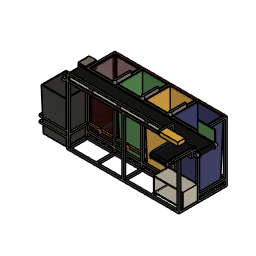
e-waste v4 ATOM (Autodesk Fusion 360 design; units mm, degrees)
Autodesk Fusion 360 part; units mm, degrees
(part 1 of 3)
sketch "Sketch1" plane through (0, 0, 0) normal (0, 0, 1) x (1, 0, 0)
sketch "Sketch1 (2)" plane through (0, 0, 0) normal (0, 0, 1) x (1, 0, 0) in component "belt sensor"
  line L0 (1400, -450) -> (1200, -450)
  line L1 (1200, -450) -> (1200, -800)
  line L2 (1200, -800) -> (1400, -800)
  line L3 (1400, -800) -> (1400, -450)
  constraint horizontal L0
  constraint perpendicular L0 L1
  constraint perpendicular L1 L2
  constraint perpendicular L0 L3
extrude "Extrude1" add sketch "Sketch1 (2)" along normal blind 70 makes body 1 in component "belt sensor"
sketch "Sketch2" plane through (1400, 0, 0) normal (1, 0, 0) x (0, 1, 0) in component "belt sensor"
sketch "Sketch3" plane through (1400, 0, 0) normal (1, 0, 0) x (0, 1, 0) in component "belt sensor"
sketch "Sketch4" plane through (1400, 0, 0) normal (1, 0, 0) x (0, 1, 0) in component "belt sensor"
  circle A0 centre (-800, 35) radius 35
  circle A1 centre (-800, 35) radius 30
  constraint concentric A0 A1
extrude "Extrude2" add sketch "Sketch4" against normal blind 200 bodies 1 in component "belt sensor"
sketch "Sketch5" plane through (1400, 0, 0) normal (1, 0, 0) x (0, 1, 0) in component "belt sensor"
  circle A0 centre (-450, 35) radius 35
  circle A1 centre (-450, 35) radius 30
  constraint concentric A0 A1
extrude "Extrude3" add sketch "Sketch5" against normal blind 200 bodies 1 in component "belt sensor"
sketch "Sketch6" plane through (1400, 0, 0) normal (1, 0, 0) x (0, 1, 0) in component "belt sensor"
  line L0 (-800, 65) -> (-450, 65)
  line L1 (-450, 65) -> (-450, 5)
  line L2 (-450, 5) -> (-800, 5)
  line L3 (-800, 5) -> (-800, 65)
  constraint horizontal L0
  constraint vertical L1
  constraint horizontal L2
  constraint vertical L3
extrude "Extrude4" cut sketch "Sketch6" against normal blind 300 bodies 1 in component "belt sensor"
sketch "Sketch7" plane through (1400, 0, 0) normal (1, 0, 0) x (0, 1, 0) in component "belt sensor"
  line L0 (-450, 5) -> (-800, 5)
  arc A0 (-800, 65) -> (-800, 5) centre (-800, 35) ccw
  line L1 (-800, 65) -> (-450, 65)
  arc A1 (-450, 5) -> (-450, 65) centre (-450, 35) ccw
  arc A2 (-450, 0) -> (-450, 70) centre (-450, 35) ccw
  line L2 (-450, 70) -> (-800, 70)
  arc A3 (-800, 70) -> (-800, 0) centre (-800, 35) ccw
  line L3 (-800, 0) -> (-450, 0)
  circle A4 centre (-800, 35) radius 27.5
  dimension "d42" = 55
  constraint concentric A0 A4
  measures "d42" diameter of A4
extrude "Extrude5" add sketch "Sketch7" against normal blind 200 separate body contours A4 makes body 2 in component "belt sensor"
sketch "Sketch8" plane through (1400, 0, 0) normal (1, 0, 0) x (0, 1, 0) in component "belt sensor"
  circle A0 centre (-800, 35) radius 27.5
  circle A1 centre (-450, 35) radius 27.5
  dimension "d45" = 55
  measures "d45" diameter of A1
extrude "Extrude6" add sketch "Sketch8" against normal blind 200 separate body contours A1 makes body 3 in component "belt sensor"
move_body "Move1" bodies 2 3 1 to x (1, 0, 0) y (0, 1, 0) z (0, 0, 1) at (0, 180, 750) in component "belt sensor"
move_body "Move2" bodies 2 3 1 to x (1, 0, 0) y (0, 1, 0) z (0, 0, 1) at (200, 0, 0) in component "belt sensor"
sketch "Sketch1 (3)" plane through (0, 0, 0) normal (0, 1, 0) x (1, 0, 0) in component "belt"
  line L0 (0, 500) -> (1800, 500)
  line L1 (1800, 500) -> (1800, 430)
  line L2 (1800, 430) -> (0, 430)
  line L3 (0, 430) -> (0, 500)
  dimension "d68" = 1800
  dimension "d69" = 70
  constraint horizontal L0
  constraint perpendicular L0 L1
  constraint perpendicular L1 L2
  constraint perpendicular L0 L3
  measures "d68" distance of L0.start L0.end
  measures "d69" distance of L0.end L1.end
extrude "Extrude1'" add sketch "Sketch1 (3)" along normal blind 200 separate body makes body 4 in component "belt"
sketch "Sketch2 (2)" plane through (0, 0, 0) normal (0, -1, 0) x (1, 0, 0) in component "belt"
  line L0 (1800, -430) -> (0, -430)
  line L1 (0, -430) -> (0, -500)
  line L2 (0, -500) -> (1800, -500)
  line L3 (1800, -500) -> (1800, -430)
  circle A0 centre (0, -465) radius 35
  circle A1 centre (0, -465) radius 30
  dimension "d72" = 60
  constraint midpoint L1 A0.centre
  constraint coincident L0.end A0
  constraint concentric A0 A1
  measures "d72" diameter of A1
extrude "Extrude2'" add sketch "Sketch2 (2)" against normal blind 200 contours L1 A0 A1 picked at (-12.8396, -434.3307) bodies 4 in component "belt"
sketch "Sketch3 (2)" plane through (0, 0, 0) normal (0, -1, 0) x (1, 0, 0) in component "belt"
  line L0 (0, -500) -> (1800, -500)
  line L1 (1800, -500) -> (1800, -430)
  line L2 (1800, -430) -> (0, -430)
  arc A0 (0, -430) -> (0, -500) centre (0, -465) ccw
  arc A1 (0, -435) -> (0, -495) centre (0, -465) ccw
  line L3 (0, -435) -> (0, -495)
  circle A2 centre (1800, -465) radius 35
  circle A3 centre (1800, -465) radius 30
  dimension "d75" = 60
  constraint midpoint L1 A2.centre
  constraint coincident L1.end A2
  constraint concentric A2 A3
  measures "d75" diameter of A3
extrude "Extrude3'" add sketch "Sketch3 (2)" against normal blind 200 contours L1 A2 A3 picked at (1831.4014, -454.0493) bodies 4 in component "belt"
sketch "Sketch4 (2)" plane through (0, 0, 0) normal (0, -1, 0) x (1, 0, 0) in component "belt"
  line L0 (1800, -430) -> (0, -430)
  arc A0 (0, -430) -> (0, -500) centre (0, -465) ccw
  line L1 (0, -500) -> (1800, -500)
  arc A1 (1800, -500) -> (1800, -430) centre (1800, -465) ccw
  arc A2 (1800, -495) -> (1800, -435) centre (1800, -465) ccw
  line L2 (1800, -495) -> (1800, -435)
  arc A3 (0, -435) -> (0, -495) centre (0, -465) ccw
  line L3 (0, -435) -> (0, -495)
  line L4 (0, -435) -> (1800, -435)
  line L5 (1800, -435) -> (1800, -495)
  line L6 (1800, -495) -> (0, -495)
  line L7 (0, -495) -> (0, -435)
  constraint horizontal L4
  constraint vertical L5
  constraint horizontal L6
  constraint vertical L7
  constraint coincident A2.start L2.start
  constraint coincident A3.start L3.start
extrude "Extrude4'" cut sketch "Sketch4 (2)" against normal blind 300 contours L2 L3 L4 L5 L6 L7 bodies 4 in component "belt"
sketch "Sketch5 (2)" plane through (0, 0, 0) normal (0, -1, 0) x (1, 0, 0) in component "belt"
  line L0 (0, -435) -> (1800, -435)
  arc A0 (1800, -495) -> (1800, -435) centre (1800, -465) ccw
  line L1 (1800, -495) -> (0, -495)
  arc A1 (0, -435) -> (0, -495) centre (0, -465) ccw
  line L2 (1800, -430) -> (0, -430)
  arc A2 (0, -430) -> (0, -500) centre (0, -465) ccw
  line L3 (0, -500) -> (1800, -500)
  arc A3 (1800, -500) -> (1800, -430) centre (1800, -465) ccw
  circle A4 centre (0, -465) radius 27.5
  circle A5 centre (1800, -465) radius 27.5
  dimension "d80" = 55
  dimension "d81" = 55
  constraint concentric A1 A4
  constraint concentric A0 A5
  measures "d80" diameter of A4
  measures "d81" diameter of A5
extrude "Extrude5'" add sketch "Sketch5 (2)" against normal blind 200 separate body contours A4 | A5 makes body 5 at (27.3633, 66.6667, -467.7381) makes body 6 at (1816.053, 133.3333, -442.6717) in component "belt"
move_body "Move1'" bodies 5 4 6 to x (1, 0, 0) y (0, 1, 0) z (0, 0, 1) at (0, -225, 1250) in component "belt"
move_body "Move2'" bodies 5 4 6 to x (1, 0, 0) y (0, 1, 0) z (0, 0, 1) at (-160, 0, 0) in component "belt"
sketch "Sketch1 (4)" plane through (0, 0, 0) normal (0, 1, 0) x (1, 0, 0) in component "power"
  line L0 (1500, 0) -> (1100, 0)
  line L1 (1100, 0) -> (1100, -200)
  line L2 (1100, -200) -> (1500, -200)
  line L3 (1500, -200) -> (1500, 0)
  dimension "d313" = 400
  constraint horizontal L0
  constraint perpendicular L0 L1
  constraint perpendicular L1 L2
  constraint perpendicular L0 L3
  measures "d313" distance of L1 L3
extrude "Extrude1''" add sketch "Sketch1 (4)" against normal blind 200 separate body makes body 7 in component "power"
sketch "Sketch2 (3)" plane through (0, -200, 0) normal (0, -1, 0) x (1, 0, 0) in component "power"
  line L0 (1500, 0) -> (1500, 200)
  line L1 (1500, 200) -> (1100, 200)
  line L2 (1100, 200) -> (1100, 0)
  line L3 (1100, 0) -> (1500, 0)
  line L4 (1110, 190) -> (1490, 190)
  line L5 (1490, 190) -> (1490, 10)
  line L6 (1490, 10) -> (1110, 10)
  line L7 (1110, 10) -> (1110, 190)
  dimension "d314" = 10
  dimension "d315" = 10
  dimension "d316" = 10
  dimension "d317" = 10
  constraint perpendicular L0 L4
  constraint perpendicular L4 L5
  constraint perpendicular L5 L6
  constraint perpendicular L4 L7
  measures "d314" distance of L0 L5
  measures "d315" distance of L2 L7
  measures "d316" distance of L1 L4
  measures "d317" distance of L3 L6
extrude "Extrude2''" cut sketch "Sketch2 (3)" against normal blind 190 contours L4 L5 L6 L7 bodies 7 in component "power"
sketch "Sketch2 (4)" plane through (0, 0, 0) normal (0, 0, 1) x (1, 0, 0)
sketch "Sketch1 (5)" plane through (0, 0, 0) normal (0, 0, 1) x (1, 0, 0) in component "vibrator"
  line L0 (0, 850) -> (200, 850)
  line L1 (200, 850) -> (200, 1050)
  line L2 (200, 1050) -> (0, 1050)
  line L3 (0, 1050) -> (0, 850)
  dimension "d89" = 200
  dimension "d90" = 200
  constraint horizontal L0
  constraint perpendicular L0 L1
  constraint perpendicular L1 L2
  constraint perpendicular L0 L3
  measures "d89" distance of L0.start L0.end
  measures "d90" distance of L0.end L1.end
sketch "Sketch1 (6)" plane through (0, 0, 0) normal (0, 0, 1) x (1, 0, 0) in component "bin case"
  line L0 (-109.9325, 100) -> (-459.9325, 100)
  line L1 (-459.9325, 100) -> (-459.9325, 450)
  line L2 (-459.9325, 450) -> (-109.9325, 450)
  line L3 (-109.9325, 450) -> (-109.9325, 100)
  line L4 (-84.9325, 450) -> (265.0675, 450)
  line L5 (265.0675, 450) -> (265.0675, 100)
  line L6 (265.0675, 100) -> (-84.9325, 100)
  line L7 (-84.9325, 100) -> (-84.9325, 450)
  line L8 (-84.9325, 100) -> (-84.9325, 450)
  line L9 (290.0675, 450) -> (640.0675, 450)
  line L10 (640.0675, 450) -> (640.0675, 100)
  line L11 (640.0675, 100) -> (290.0675, 100)
  line L12 (290.0675, 100) -> (290.0675, 450)
  line L13 (665.0675, 450) -> (1015.0675, 450)
  line L14 (1015.0675, 450) -> (1015.0675, 100)
  line L15 (1015.0675, 100) -> (665.0675, 100)
  line L16 (665.0675, 100) -> (665.0675, 450)
  line L17 (-484.9325, 475) -> (1040.0675, 475)
  line L18 (1040.0675, 475) -> (1040.0675, 75)
  line L19 (1040.0675, 75) -> (-484.9325, 75)
  line L20 (-484.9325, 75) -> (-484.9325, 475)
  dimension "d101" = 350
  dimension "d102" = 350
  dimension "d103" = 350
  dimension "d104" = 25
  dimension "d105" = 25
  dimension "d106" = 25
  dimension "d107" = 350
  dimension "d108" = 350
  dimension "d109" = 25
  dimension "d110" = 25
  dimension "d111" = 25
  dimension "d112" = 25
  constraint horizontal L0
  constraint vertical L1
  constraint horizontal L2
  constraint vertical L3
  constraint horizontal L4
  constraint vertical L5
  constraint horizontal L6
  constraint vertical L7
  constraint vertical L8
  constraint horizontal L9
  constraint vertical L10
  constraint horizontal L11
  constraint vertical L12
  constraint horizontal L13
  constraint vertical L14
  constraint horizontal L15
  constraint vertical L16
  constraint horizontal L17
  constraint vertical L18
  constraint horizontal L19
  constraint vertical L20
  measures "d101" distance of L0.start L0.end
  measures "d102" distance of L5.end L6.end
  measures "d103" distance of L10.end L11.end
  measures "d104" distance of L5 L12
  measures "d105" distance of L3 L7
  measures "d106" distance of L10 L16
  measures "d107" distance of L14.end L15.end
  measures "d108" distance of L0.end L1.end
  measures "d109" distance of L1 L20
  measures "d110" distance of L14 L18
  measures "d111" distance of L13 L17
  measures "d112" distance of L15 L19
extrude "Extrude1'''" add sketch "Sketch1 (6)" along normal blind 25 separate body makes body 8 in component "bin case"
sketch "Sketch1 (7)" plane through (0, 0, 0) normal (0, 0, 1) x (1, 0, 0) in component "bin case (1)"
  line L0 (-109.9325, 100) -> (-459.9325, 100)
  line L1 (-459.9325, 100) -> (-459.9325, 450)
  line L2 (-459.9325, 450) -> (-109.9325, 450)
  line L3 (-109.9325, 450) -> (-109.9325, 100)
  line L4 (-84.9325, 450) -> (265.0675, 450)
  line L5 (265.0675, 450) -> (265.0675, 100)
  line L6 (265.0675, 100) -> (-84.9325, 100)
  line L7 (-84.9325, 100) -> (-84.9325, 450)
  line L8 (-84.9325, 100) -> (-84.9325, 450)
  line L9 (290.0675, 450) -> (640.0675, 450)
  line L10 (640.0675, 450) -> (640.0675, 100)
  line L11 (640.0675, 100) -> (290.0675, 100)
  line L12 (290.0675, 100) -> (290.0675, 450)
  line L13 (665.0675, 450) -> (1015.0675, 450)
  line L14 (1015.0675, 450) -> (1015.0675, 100)
  line L15 (1015.0675, 100) -> (665.0675, 100)
  line L16 (665.0675, 100) -> (665.0675, 450)
  line L17 (-484.9325, 475) -> (1040.0675, 475)
  line L18 (1040.0675, 475) -> (1040.0675, 75)
  line L19 (1040.0675, 75) -> (-484.9325, 75)
  line L20 (-484.9325, 75) -> (-484.9325, 475)
  dimension "d101_1" = 350
  dimension "d102_1" = 350
  dimension "d103_1" = 350
  dimension "d104_1" = 25
  dimension "d105_1" = 25
  dimension "d106_1" = 25
  dimension "d107_1" = 350
  dimension "d108_1" = 350
  dimension "d109_1" = 25
  dimension "d110_1" = 25
  dimension "d111_1" = 25
  dimension "d112_1" = 25
  constraint horizontal L0
  constraint vertical L1
  constraint horizontal L2
  constraint vertical L3
  constraint horizontal L4
  constraint vertical L5
  constraint horizontal L6
  constraint vertical L7
  constraint vertical L8
  constraint horizontal L9
  constraint vertical L10
  constraint horizontal L11
  constraint vertical L12
  constraint horizontal L13
  constraint vertical L14
  constraint horizontal L15
  constraint vertical L16
  constraint horizontal L17
  constraint vertical L18
  constraint horizontal L19
  constraint vertical L20
  measures "d101_1" distance of L0.start L0.end
  measures "d102_1" distance of L5.end L6.end
  measures "d103_1" distance of L10.end L11.end
  measures "d104_1" distance of L5 L12
  measures "d105_1" distance of L3 L7
  measures "d106_1" distance of L10 L16
  measures "d107_1" distance of L14.end L15.end
  measures "d108_1" distance of L0.end L1.end
  measures "d109_1" distance of L1 L20
  measures "d110_1" distance of L14 L18
  measures "d111_1" distance of L13 L17
  measures "d112_1" distance of L15 L19
extrude "Extrude1''''" add sketch "Sketch1 (7)" along normal blind 25 separate body makes body 9 in component "bin case (1)"
sketch "Sketch3 (3)" plane through (0, 0, 25) normal (0, 0, 1) x (-1, 0, 0)
  line L0 (-265.0675, -100) -> (84.9325, -100)
  line L1 (84.9325, -100) -> (84.9325, -450)
  line L2 (84.9325, -450) -> (-265.0675, -450)
  line L3 (-265.0675, -450) -> (-265.0675, -100)
  line L4 (459.9325, -450) -> (109.9325, -450)
  line L5 (109.9325, -450) -> (109.9325, -100)
  line L6 (109.9325, -100) -> (459.9325, -100)
  line L7 (459.9325, -100) -> (459.9325, -450)
  line L8 (-640.0675, -100) -> (-290.0675, -100)
  line L9 (-290.0675, -100) -> (-290.0675, -450)
  line L10 (-290.0675, -450) -> (-640.0675, -450)
  line L11 (-640.0675, -450) -> (-640.0675, -100)
  line L12 (-1015.0675, -100) -> (-665.0675, -100)
  line L13 (-665.0675, -100) -> (-665.0675, -450)
  line L14 (-665.0675, -450) -> (-1015.0675, -450)
  line L15 (-1015.0675, -450) -> (-1015.0675, -100)
  line L16 (484.9325, -75) -> (-1040.0675, -75)
  line L17 (-1040.0675, -75) -> (-1040.0675, -475)
  line L18 (-1040.0675, -475) -> (484.9325, -475)
  line L19 (484.9325, -475) -> (484.9325, -75)
  line L20 (459.9325, -450) -> (484.9325, -450)
  line L21 (484.9325, -450) -> (484.9325, -475)
  line L22 (484.9325, -475) -> (459.9325, -475)
  line L23 (459.9325, -475) -> (459.9325, -450)
  line L24 (84.9325, -450) -> (109.9325, -450)
  line L25 (109.9325, -450) -> (109.9325, -475)
  line L26 (84.9325, -475) -> (84.9325, -450)
  line L27 (109.9325, -475) -> (84.9325, -475)
  line L28 (-290.0675, -450) -> (-265.0675, -450)
  line L29 (-265.0675, -450) -> (-265.0675, -475)
  line L30 (-290.0675, -475) -> (-290.0675, -450)
  line L31 (-265.0675, -475) -> (-290.0675, -475)
  line L32 (-665.0675, -450) -> (-640.0675, -450)
  line L33 (-640.0675, -450) -> (-640.0675, -475)
  line L34 (-665.0675, -475) -> (-665.0675, -450)
  line L35 (-640.0675, -475) -> (-665.0675, -475)
  line L36 (-1040.0675, -450) -> (-1015.0675, -450)
  line L37 (-1015.0675, -450) -> (-1015.0675, -475)
  line L38 (-1040.0675, -475) -> (-1040.0675, -450)
  line L39 (-1015.0675, -475) -> (-1040.0675, -475)
  line L40 (459.9325, -75) -> (484.9325, -75)
  line L41 (484.9325, -75) -> (484.9325, -100)
  line L42 (459.9325, -100) -> (459.9325, -75)
  line L43 (484.9325, -100) -> (459.9325, -100)
  line L44 (84.9325, -75) -> (109.9325, -75)
  line L45 (109.9325, -75) -> (109.9325, -100)
  line L46 (84.9325, -100) -> (84.9325, -75)
  line L47 (109.9325, -100) -> (84.9325, -100)
  line L48 (-290.0675, -75) -> (-265.0675, -75)
  line L49 (-265.0675, -75) -> (-265.0675, -100)
  line L50 (-290.0675, -100) -> (-290.0675, -75)
  line L51 (-265.0675, -100) -> (-290.0675, -100)
  line L52 (-665.0675, -75) -> (-640.0675, -75)
  line L53 (-640.0675, -75) -> (-640.0675, -100)
  line L54 (-665.0675, -100) -> (-665.0675, -75)
  line L55 (-640.0675, -100) -> (-665.0675, -100)
  line L56 (-1040.0675, -75) -> (-1015.0675, -75)
  line L57 (-1015.0675, -75) -> (-1015.0675, -100)
  line L58 (-1040.0675, -100) -> (-1040.0675, -75)
  line L59 (-1015.0675, -100) -> (-1040.0675, -100)
  dimension "d117" = -1500
  dimension "d118" = 375
  constraint horizontal L20
  constraint vertical L21
  constraint horizontal L22
  constraint vertical L23
  constraint coincident L18.end L19.start
  constraint coincident L4.start L7.end
move_body "Move1''" bodies 8 to x (1, 0, 0) y (0, 1, 0) z (0, 0, 1) at (0, 0, 800) in component "bin case"
extrude "Extrude2'''" add sketch "Sketch3 (3)" along normal blind 775 contours L16 L48 L49 L50 L51 | L16 L44 L45 L46 L47 | L18 L28 L29 L30 L31 | L18 L24 L25 L26 L27 | L16 L52 L53 L54 L55 | L16 L19 L40 L41 L42 L43 | L18 L32 L33 L34 L35 | L18 L19 L20 L21 L22 L23 | L16 L17 L56 L57 L58 L59 | L17 L18 L36 L37 L38 L39 bodies 8 in component "bin case"
combine "Combine1" operation add target body 9 tool bodies 8 in component "bin case (1)"
sketch "Sketch4 (3)" plane through (-459.9325, 0, 0) normal (1, 0, 0) x (0, 1, 0)
  line L0 (100, 0) -> (450, 0)
  line L1 (450, 0) -> (450, 25)
  line L2 (450, 25) -> (100, 25)
  line L3 (100, 25) -> (100, 0)
sketch "Sketch5 (3)" plane through (-459.9325, 275, 12.5) normal (1, 0, 0) x (0, 1, 0)
sketch "Sketch6 (2)" plane through (1040.0675, 0, 0) normal (1, 0, 0) x (0, 1, 0)
  line L0 (75, 825) -> (75, 0)
  line L1 (75, 0) -> (475, 0)
  line L2 (475, 0) -> (475, 825)
  line L3 (475, 825) -> (75, 825)
  line L4 (100, 25) -> (100, 800)
  line L5 (100, 800) -> (450, 800)
  line L6 (450, 800) -> (450, 25)
  line L7 (450, 25) -> (100, 25)
  line L8 (200, 25) -> (225, 25)
  line L9 (225, 25) -> (225, 0)
  line L10 (225, 0) -> (200, 0)
  line L11 (200, 0) -> (200, 25)
  line L12 (325, 25) -> (350, 25)
  line L13 (350, 25) -> (350, 0)
  line L14 (350, 0) -> (325, 0)
  line L15 (325, 0) -> (325, 25)
  dimension "d121" = 25
  dimension "d122" = 25
  dimension "d123" = 100
  dimension "d124" = 100
  constraint horizontal L8
  constraint vertical L9
  constraint horizontal L10
  constraint vertical L11
  constraint coincident L7 L8.start
  constraint horizontal L12
  constraint vertical L13
  constraint horizontal L14
  constraint vertical L15
  constraint coincident L7 L12.start
  measures "d121" distance of L8.start L8.end
  measures "d122" distance of L12.start L12.end
  measures "d123" distance of L4 L11
  measures "d124" distance of L6 L13
extrude "Extrude2''''" add sketch "Sketch6 (2)" against normal blind 1525 contours L1 L7 L8 L9 L10 L11 | L1 L7 L12 L13 L14 L15 bodies 9 in component "bin case (1)"
sketch "Sketch7 (2)" plane through (0, 75, 0) normal (0, -1, 0) x (1, 0, 0)
  line L0 (1015.0675, 25) -> (665.0675, 25)
  line L1 (665.0675, 25) -> (665.0675, 800)
  line L2 (665.0675, 800) -> (1015.0675, 800)
  line L3 (1015.0675, 800) -> (1015.0675, 25)
  line L4 (265.0675, 25) -> (-84.9325, 25)
  line L5 (-84.9325, 25) -> (-84.9325, 800)
  line L6 (-84.9325, 800) -> (265.0675, 800)
  line L7 (265.0675, 800) -> (265.0675, 25)
  line L8 (1040.0675, 0) -> (1040.0675, 825)
  line L9 (1040.0675, 825) -> (-484.9325, 825)
  line L10 (-484.9325, 825) -> (-484.9325, 0)
  line L11 (-484.9325, 0) -> (1040.0675, 0)
  line L12 (-459.9325, 25) -> (-459.9325, 800)
  line L13 (-459.9325, 800) -> (-109.9325, 800)
  line L14 (-109.9325, 800) -> (-109.9325, 25)
  line L15 (-109.9325, 25) -> (-459.9325, 25)
  line L16 (290.0675, 25) -> (290.0675, 800)
  line L17 (290.0675, 800) -> (640.0675, 800)
  line L18 (640.0675, 800) -> (640.0675, 25)
  line L19 (640.0675, 25) -> (290.0675, 25)
sketch "Sketch8 (2)" plane through (0, 75, 0) normal (0, -1, 0) x (1, 0, 0)
  line L0 (-485, 875) -> (-585, 875)
  line L1 (-585, 875) -> (-585, 775)
  line L2 (-585, 775) -> (-485, 775)
  line L3 (-485, 775) -> (-485, 875)
  line L4 (1040.0675, 825) -> (-484.9325, 825)
  line L5 (-575, 865) -> (-495, 865)
  line L6 (-495, 865) -> (-495, 785)
  line L7 (-495, 785) -> (-575, 785)
  line L8 (-575, 785) -> (-575, 865)
  dimension "d133" = 100
  dimension "d134" = 100
  dimension "d135" = 50
  dimension "d136" = 10
  dimension "d137" = 10
  dimension "d138" = 10
  dimension "d139" = 10
  constraint horizontal L0
  constraint vertical L1
  constraint horizontal L2
  constraint vertical L3
  constraint horizontal L5
  constraint vertical L6
  constraint horizontal L7
  constraint vertical L8
  measures "d133" distance of L0.start L0.end
  measures "d134" distance of L0.end L1.end
  measures "d135" distance of L0 L4
  measures "d136" distance of L1 L8
  measures "d137" distance of L3 L6
  measures "d138" distance of L2 L7
  measures "d139" distance of L0 L5
extrude "Extrude1'''''" add sketch "Sketch8 (2)" against normal blind 150 separate body makes body 10
copy_body "CutPasteBodies1" bodies 10 removing the originals makes body 11 in component "motor belt"
sketch "Sketch1 (8)" plane through (0, 75, 0) normal (0, -1, 0) x (1, 0, 0) in component "motor belt"
  line L0 (-495, 785) -> (-575, 785)
  line L1 (-575, 785) -> (-575, 865)
  line L2 (-575, 865) -> (-495, 865)
  line L3 (-495, 865) -> (-495, 785)
  line L4 (-485, 775) -> (-485, 875)
  line L5 (-485, 875) -> (-585, 875)
  line L6 (-585, 875) -> (-585, 775)
  line L7 (-585, 775) -> (-485, 775)
  circle A0 centre (-535, 825) radius 40
  constraint tangent L0 A0
extrude "Extrude1''''''" add sketch "Sketch1 (8)" against normal blind 100 separate body contours A0 makes body 12 in component "motor belt"
sketch "Sketch2 (5)" plane through (0, 75, 0) normal (0, -1, 0) x (1, 0, 0) in component "motor belt"
  circle A0 centre (-535, 825) radius 40
  circle A1 centre (-535, 825) radius 20
  dimension "d144" = 40
  constraint concentric A0 A1
  measures "d144" diameter of A1
extrude "Extrude2'''''" add sketch "Sketch2 (5)" along normal blind 20 contours A1 bodies 12 in component "motor belt"
move_body "Move1'''" bodies 12 11 to x (1, 0, 0) y (0, 1, 0) z (0, 0, 1) at (0, 0, -30) in component "motor belt"
sketch "Sketch9" plane through (1040.0675, 0, 0) normal (1, 0, 0) x (0, 1, 0)
  line L0 (450, 25) -> (100, 25)
  line L1 (100, 25) -> (100, 800)
  line L2 (100, 800) -> (450, 800)
  line L3 (450, 800) -> (450, 25)
  line L4 (75, 0) -> (475, 0)
  line L5 (475, 0) -> (475, 825)
  line L6 (475, 825) -> (75, 825)
  line L7 (75, 825) -> (75, 0)
  line L8 (100, 800) -> (75, 800)
  line L9 (75, 800) -> (75, 825)
  line L10 (75, 825) -> (100, 825)
  line L11 (100, 825) -> (100, 800)
  constraint horizontal L8
  constraint vertical L9
  constraint horizontal L10
  constraint vertical L11
  constraint coincident L6.end L7.start
  constraint coincident L1.end L2.start
extrude "Extrude3''" add sketch "Sketch9" along normal blind 180 contours L6 L7 L8 L9 L10 L11 bodies 9 in component "bin case (1)"
sketch "Sketch10" plane through (0, 100, 0) normal (0, 1, 0) x (-1, 0, 0)
  line L0 (-1040.0675, 800) -> (-1040.0675, 825)
  line L1 (-1040.0675, 825) -> (-1220.0675, 825)
  line L2 (-1220.0675, 825) -> (-1220.0675, 800)
  line L3 (-1220.0675, 800) -> (-1040.0675, 800)
  circle A0 centre (-1265, 795) radius 27.5
  circle A1 centre (-1265, 795) radius 20
  dimension "d165" = 40
  constraint concentric A0 A1
  measures "d165" diameter of A1
extrude "Extrude2''''''" add sketch "Sketch10" against normal blind 45 separate body contours A1 makes body 13
copy_body "CutPasteBodies1'" bodies 13 removing the originals makes body 14 in component "bin case (1)"
sketch "Sketch11" plane through (0, 100, 0) normal (0, 1, 0) x (-1, 0, 0)
  line L0 (-1040.0675, 800) -> (-1040.0675, 825)
  line L1 (-1040.0675, 825) -> (-1220.0675, 825)
  line L2 (-1220.0675, 825) -> (-1220.0675, 800)
  line L3 (-1220.0675, 800) -> (-1040.0675, 800)
  line L4 (-1220.0675, 800) -> (-1255.8504, 780.0908)
  line L5 (-1220.0675, 825) -> (-1255.8504, 805.0908)
  line L6 (-1255.8504, 805.0908) -> (-1255.8504, 780.0908)
  constraint coincident L2.end L3.start
  constraint coincident L1.end L2.start
  constraint parallel L4 L5
extrude "Extrude4''" add sketch "Sketch11" against normal blind 25 contours L2 L4 L5 L6 bodies 9 14 in component "bin case (1)"
sketch "Sketch12" plane through (0, 75, 0) normal (0, -1, 0) x (1, 0, 0)
  line L0 (1015.0675, 25) -> (665.0675, 25)
  line L1 (665.0675, 25) -> (665.0675, 800)
  line L2 (665.0675, 800) -> (1015.0675, 800)
  line L3 (1015.0675, 800) -> (1015.0675, 25)
  line L4 (265.0675, 25) -> (-84.9325, 25)
  line L5 (-84.9325, 25) -> (-84.9325, 800)
  line L6 (-84.9325, 800) -> (265.0675, 800)
  line L7 (265.0675, 800) -> (265.0675, 25)
  line L8 (1040.0675, 0) -> (1040.0675, 800)
  line L9 (1040.0675, 800) -> (1220.0675, 800)
  line L10 (1220.0675, 800) -> (1248.0054, 784.4556)
  arc A0 (1250.0695, 808.3072) -> (1248.0054, 784.4556) centre (1265, 795) ccw
  line L11 (1250.0695, 808.3072) -> (1220.0675, 825)
  line L12 (1220.0675, 825) -> (-484.9325, 825)
  line L13 (-484.9325, 825) -> (-484.9325, 0)
  line L14 (-484.9325, 0) -> (1040.0675, 0)
  line L15 (-459.9325, 25) -> (-459.9325, 800)
  line L16 (-459.9325, 800) -> (-109.9325, 800)
  line L17 (-109.9325, 800) -> (-109.9325, 25)
  line L18 (-109.9325, 25) -> (-459.9325, 25)
  line L19 (290.0675, 25) -> (290.0675, 800)
  line L20 (290.0675, 800) -> (640.0675, 800)
  line L21 (640.0675, 800) -> (640.0675, 25)
  line L22 (640.0675, 25) -> (290.0675, 25)
ref_plane "WorkPlane1" through (382.5685, -145, 412.5) normal (0, -1, 0) x (1, 0, 0)
sketch "Sketch13" plane through (0, -145, 0) normal (0, -1, 0) x (-1, 0, 0)
  line L0 (460, -800) -> (-1220, -800)
  line L1 (-1220, -800) -> (-1265, -775)
  line L2 (-1220, -825) -> (-1265, -800)
  line L3 (-1265, -800) -> (-1265, -775)
  line L4 (-1220, -825) -> (486, -825)
  line L5 (486, -825) -> (486, -800)
  line L6 (486, -800) -> (460, -800)
  circle A0 centre (-1265, -795) radius 20
  constraint horizontal L0
  constraint parallel L1 L2
  constraint vertical L3
  constraint perpendicular L3 L4
  constraint perpendicular L4 L5
  constraint perpendicular L5 L6
  constraint coincident L1.end A0
extrude "Extrude3'''" add sketch "Sketch13" along normal blind 25 separate body makes body 15
copy_body "CutPasteBodies2" bodies 15 removing the originals makes body 16 in component "bin case (1)"
move_body "Move1''''" bodies 16 to x (1, 0, 0) y (0, 1, 0) z (0, 0, 1) at (0, -20, 0) in component "bin case (1)"
move_body "Move2''" bodies 16 to x (1, 0, 0) y (0, 1, 0) z (0, 0, 1) at (0, 10, 0) in component "bin case (1)"
sketch "Sketch14" plane through (0, -155, 0) normal (0, 1, 0) x (-1, 0, 0)
  line L0 (486, 825) -> (-1220, 825)
  line L1 (-1220, 825) -> (-1250.0621, 808.2988)
  arc A0 (-1250.0621, 808.2988) -> (-1248.0189, 784.434) centre (-1265, 795) ccw
  line L2 (-1248.0189, 784.434) -> (-1220, 800)
  line L3 (-1220, 800) -> (486, 800)
  line L4 (486, 800) -> (486, 825)
  circle A1 centre (-1265, 795) radius 20
  circle A2 centre (-1265, 795) radius 20
  circle A3 centre (-1265, 795) radius 20
  circle A4 centre (-1265, 795) radius 20
extrude "Extrude5''" add sketch "Sketch14" along normal blind 10 contours A0 A1 A2 A3 A4 bodies 16 in component "bin case (1)"
sketch "Sketch15" plane through (0, -180, 0) normal (0, -1, 0) x (1, 0, 0)
  line L0 (1220, 825) -> (-486, 825)
  line L1 (-486, 825) -> (-486, 800)
  line L2 (-486, 800) -> (1220, 800)
  line L3 (1220, 800) -> (1248.0189, 784.434)
  arc A0 (1248.0189, 784.434) -> (1250.0621, 808.2988) centre (1265, 795) ccw
  line L4 (1250.0621, 808.2988) -> (1220, 825)
  circle A1 centre (-534.95, 795) radius 27.5
  circle A2 centre (-534.95, 795) radius 20
  dimension "d175" = 40
  constraint concentric A1 A2
  measures "d175" diameter of A2
extrude "Extrude4'''" add sketch "Sketch15" against normal blind 35 separate body contours A2 makes body 17
sketch "Sketch16" plane through (0, -180, 0) normal (0, -1, 0) x (1, 0, 0)
  line L0 (1220, 825) -> (-486, 825)
  line L1 (-486, 825) -> (-486, 800)
  line L2 (-486, 800) -> (1220, 800)
  line L3 (1220, 800) -> (1248.0189, 784.434)
  arc A0 (1248.0189, 784.434) -> (1250.0621, 808.2988) centre (1265, 795) ccw
  line L4 (1250.0621, 808.2988) -> (1220, 825)
  line L5 (-486, 800) -> (-535, 775)
  line L6 (-486, 825) -> (-535, 800)
  line L7 (-535, 800) -> (-535, 775)
  constraint coincident L1.end L2.start
  constraint coincident L0.end L1.start
  constraint parallel L5 L6
  constraint parallel L1 L7
extrude "Extrude5'''" add sketch "Sketch16" against normal blind 25 contours L1 L5 L6 L7 bodies 17
copy_body "CutPasteBodies3" bodies 17 removing the originals makes body 18 in component "bin case (1)"
combine "Combine2" operation add target body 18 tool bodies 16 in component "bin case (1)"
sketch "Sketch17" plane through (0, 0, 800) normal (0, 0, -1) x (1, 0, 0)
  line L0 (-486, 155) -> (1220, 155)
  line L1 (1220, 155) -> (1220, 180)
  line L2 (1220, 180) -> (-486, 180)
  line L3 (-486, 180) -> (-486, 155)
  line L4 (-110, -100) -> (-110, 180)
  line L5 (-110, 180) -> (-85, 180)
  line L6 (-85, 180) -> (-85, 155)
  line L7 (-85, 155) -> (-110, 155)
  line L8 (-110, 155) -> (-110, 180)
  line L9 (290, 180) -> (290, 155)
  line L10 (265, 180) -> (290, 180)
  line L11 (265, 155) -> (265, 180)
  line L12 (290, 155) -> (265, 155)
  line L13 (665, 180) -> (665, 155)
  line L14 (640, 180) -> (665, 180)
  line L15 (640, 155) -> (640, 180)
  line L16 (665, 155) -> (640, 155)
  line L17 (1040, 180) -> (1040, 155)
  line L18 (1015, 180) -> (1040, 180)
  line L19 (1015, 155) -> (1015, 180)
  line L20 (1040, 155) -> (1015, 155)
  line L21 (-460, 180) -> (-460, 155)
  line L22 (-485, 180) -> (-460, 180)
  line L23 (-485, 155) -> (-485, 180)
  line L24 (-460, 155) -> (-485, 155)
  dimension "d181" = 25
  dimension "d184" = 1125
  dimension "d185" = 0
  dimension "d188" = -375
  dimension "d189" = 0
  constraint coincident L2 L4.end
  constraint perpendicular L2 L4
  constraint horizontal L5
  constraint vertical L6
  constraint horizontal L7
  constraint vertical L8
  constraint coincident L0 L6.end
  measures "d181" distance of L4 L6
extrude "Extrude6'" add sketch "Sketch17" along normal blind 800 contours L0 L2 L21 L22 L23 L24 | L0 L2 L4 L5 L6 L7 L8 | L0 L2 L9 L10 L11 L12 | L0 L2 L13 L14 L15 L16 | L0 L2 L17 L18 L19 L20 bodies 18 in component "bin case (1)"
sketch "Sketch18" plane through (-485, 0, 0) normal (-1, 0, 0) x (0, -1, 0)
  line L0 (180, 800) -> (155, 800)
  line L1 (155, 800) -> (155, 0)
  line L2 (155, 0) -> (180, 0)
  line L3 (180, 0) -> (180, 800)
  line L4 (155, 0) -> (180, 0)
  line L5 (180, 0) -> (180, 25)
  line L6 (180, 25) -> (155, 25)
  line L7 (155, 25) -> (155, 0)
  dimension "d192" = 25
  constraint horizontal L4
  constraint vertical L5
  constraint horizontal L6
  constraint vertical L7
  constraint coincident L3 L5.end
  constraint coincident L1.end L2.start
  measures "d192" distance of L1.end L6.end
extrude "Extrude7" add sketch "Sketch18" against normal blind 1525 contours L1 L2 L3 L4 L5 L6 L7 bodies 18 in component "bin case (1)"
sketch "Sketch19" plane through (0, -180, 0) normal (0, -1, 0) x (1, 0, 0)
  line L0 (-485, 0) -> (1040, 0)
  line L1 (1040, 0) -> (1040, 800)
  line L2 (1040, 800) -> (1220, 800)
  line L3 (1220, 800) -> (1248.0189, 784.434)
  arc A0 (1248.0189, 784.434) -> (1250.0621, 808.2988) centre (1265, 795) ccw
  line L4 (1250.0621, 808.2988) -> (1220, 825)
  line L5 (1220, 825) -> (-486, 825)
  line L6 (-486, 825) -> (-519.6212, 807.8463)
  arc A1 (-519.6212, 807.8463) -> (-535, 775.0001) centre (-534.95, 795) ccw
  line L7 (-535, 775.0001) -> (-535, 775)
  line L8 (-535, 775) -> (-534.9999, 775.0001)
  arc A2 (-534.9999, 775.0001) -> (-518.7278, 783.3022) centre (-534.95, 795) ccw
  line L9 (-518.7278, 783.3022) -> (-486, 800)
  line L10 (-486, 800) -> (-485, 800)
  line L11 (-485, 800) -> (-485, 0)
  line L12 (-460, 25) -> (-460, 800)
  line L13 (-460, 800) -> (-110, 800)
  line L14 (-110, 800) -> (-110, 25)
  line L15 (-110, 25) -> (-460, 25)
  line L16 (1015, 25) -> (665, 25)
  line L17 (665, 25) -> (665, 800)
  line L18 (665, 800) -> (1015, 800)
  line L19 (1015, 800) -> (1015, 25)
  line L20 (-85, 25) -> (-85, 800)
  line L21 (-85, 800) -> (265, 800)
  line L22 (265, 800) -> (265, 25)
  line L23 (265, 25) -> (-85, 25)
  line L24 (640, 25) -> (290, 25)
  line L25 (290, 25) -> (290, 800)
  line L26 (290, 800) -> (640, 800)
  line L27 (640, 800) -> (640, 25)
  line L28 (-485, 0) -> (-460, 0)
  line L29 (-460, 0) -> (-460, 25)
  line L30 (-460, 25) -> (-485, 25)
  line L31 (-485, 25) -> (-485, 0)
  line L32 (-85, 0) -> (-85, 25)
  line L33 (-85, 25) -> (-110, 25)
  line L34 (-110, 25) -> (-110, 0)
  line L35 (-110, 0) -> (-85, 0)
  line L36 (290, 0) -> (290, 25)
  line L37 (290, 25) -> (265, 25)
  line L38 (265, 25) -> (265, 0)
  line L39 (265, 0) -> (290, 0)
  line L40 (665, 0) -> (665, 25)
  line L41 (665, 25) -> (640, 25)
  line L42 (640, 25) -> (640, 0)
  line L43 (640, 0) -> (665, 0)
  line L44 (1040, 0) -> (1040, 25)
  line L45 (1040, 25) -> (1015, 25)
  line L46 (1015, 25) -> (1015, 0)
  line L47 (1015, 0) -> (1040, 0)
  dimension "d197" = 1500
  dimension "d198" = 300
  constraint horizontal L28
  constraint vertical L29
  constraint horizontal L30
  constraint vertical L31
  constraint coincident L12.start L15.end
  constraint coincident L0.start L11.end
extrude "Extrude8" add sketch "Sketch19" against normal blind 280 contours L0 L11 L28 L29 L30 L31 | L0 L32 L33 L34 L35 | L0 L36 L37 L38 L39 | L0 L40 L41 L42 L43 | L0 L1 L44 L45 L46 L47 bodies 9 18 in component "bin case (1)"
sketch "Sketch20" plane through (0, -180, 0) normal (0, -1, 0) x (1, 0, 0)
  line L0 (1015, 25) -> (665, 25)
  line L1 (665, 25) -> (665, 800)
  line L2 (665, 800) -> (1015, 800)
  line L3 (1015, 800) -> (1015, 25)
  line L4 (640, 25) -> (290, 25)
  line L5 (290, 25) -> (290, 800)
  line L6 (290, 800) -> (640, 800)
  line L7 (640, 800) -> (640, 25)
  line L8 (-485, 0) -> (1040, 0)
  line L9 (1040, 0) -> (1040, 800)
  line L10 (1040, 800) -> (1220, 800)
  line L11 (1220, 800) -> (1248.0189, 784.434)
  arc A0 (1248.0189, 784.434) -> (1250.0621, 808.2988) centre (1265, 795) ccw
  line L12 (1250.0621, 808.2988) -> (1220, 825)
  line L13 (1220, 825) -> (-486, 825)
  line L14 (-486, 825) -> (-519.6212, 807.8463)
  arc A1 (-519.6212, 807.8463) -> (-535, 775.0001) centre (-534.95, 795) ccw
  line L15 (-535, 775.0001) -> (-535, 775)
  line L16 (-535, 775) -> (-534.9999, 775.0001)
  arc A2 (-534.9999, 775.0001) -> (-518.7278, 783.3022) centre (-534.95, 795) ccw
  line L17 (-518.7278, 783.3022) -> (-486, 800)
  line L18 (-486, 800) -> (-485, 800)
  line L19 (-485, 800) -> (-485, 0)
  line L20 (-85, 25) -> (-85, 800)
  line L21 (-85, 800) -> (265, 800)
  line L22 (265, 800) -> (265, 25)
  line L23 (265, 25) -> (-85, 25)
  line L24 (-460, 25) -> (-460, 800)
  line L25 (-460, 800) -> (-110, 800)
  line L26 (-110, 800) -> (-110, 25)
  line L27 (-110, 25) -> (-460, 25)
  line L28 (-110, 800) -> (-85, 800)
  line L29 (-85, 800) -> (-85, 25)
  line L30 (-85, 25) -> (-110, 25)
  line L31 (-110, 25) -> (-110, 800)
  line L32 (640, 800) -> (665, 800)
  line L33 (665, 800) -> (665, 25)
  line L34 (665, 25) -> (640, 25)
  line L35 (640, 25) -> (640, 800)
  constraint horizontal L28
  constraint vertical L29
  constraint horizontal L30
  constraint vertical L31
  constraint coincident L20.start L23.end
  constraint coincident L25.end L26.start
  constraint horizontal L32
  constraint vertical L33
  constraint horizontal L34
  constraint vertical L35
  constraint coincident L0.end L1.start
  constraint coincident L6.end L7.start
extrude "Extrude9" cut sketch "Sketch20" against normal blind 25 contours L1 L7 L32 L33 L34 L35 | L20 L26 L28 L29 L30 L31 bodies 9 in component "bin case (1)"
sketch "Sketch21" plane through (0, 0, 825) normal (0, 0, 1) x (-1, 0, 0)
  line L0 (-1220, 155) -> (486, 155)
  line L1 (486, 155) -> (486, 180)
  line L2 (486, 180) -> (-1220, 180)
  line L3 (-1220, 180) -> (-1220, 155)
  line L4 (460, 155) -> (485, 155)
  line L5 (485, 155) -> (485, 180)
  line L6 (485, 180) -> (460, 180)
  line L7 (460, 180) -> (460, 155)
  line L8 (-1040, 155) -> (-1015, 155)
  line L9 (-1015, 155) -> (-1015, 180)
  line L10 (-1015, 180) -> (-1040, 180)
  line L11 (-1040, 180) -> (-1040, 155)
  constraint horizontal L4
  constraint vertical L5
  constraint horizontal L6
  constraint vertical L7
  constraint coincident L2 L5.end
  constraint coincident L0 L4.start
  constraint horizontal L8
  constraint vertical L9
  constraint horizontal L10
  constraint vertical L11
  constraint coincident L2 L9.end
  constraint coincident L0 L8.start
extrude "Extrude10" add sketch "Sketch21" along normal blind 75 contours L0 L2 L8 L9 L10 L11 | L0 L2 L4 L5 L6 L7 bodies 9 in component "bin case (1)"
sketch "Sketch22" plane through (1015, 0, 0) normal (-1, 0, 0) x (0, -1, 0)
  line L0 (155, 825) -> (180, 825)
  line L1 (180, 825) -> (180, 900)
  line L2 (180, 900) -> (155, 900)
  line L3 (155, 900) -> (155, 825)
  line L4 (155, 900) -> (180, 900)
  line L5 (180, 900) -> (180, 875)
  line L6 (180, 875) -> (155, 875)
  line L7 (155, 875) -> (155, 900)
  dimension "d205" = 25
  constraint horizontal L4
  constraint vertical L5
  constraint horizontal L6
  constraint vertical L7
  constraint coincident L1 L5.end
  constraint coincident L2.end L3.start
  measures "d205" distance of L4 L6
extrude "Extrude11" add sketch "Sketch22" along normal blind 1500 contours L1 L2 L3 L4 L5 L6 L7 bodies 9 in component "bin case (1)"
sketch "Sketch23" plane through (0, 0, 900) normal (0, 0, 1) x (-1, 0, 0)
  line L0 (-1040, 180) -> (-1040, 155)
  line L1 (-1040, 155) -> (485, 155)
  line L2 (485, 155) -> (485, 180)
  line L3 (485, 180) -> (460, 180)
  line L4 (460, 180) -> (-1040, 180)
  line L5 (160, 180) -> (185, 180)
  line L6 (185, 180) -> (185, 155)
  line L7 (185, 155) -> (160, 155)
  line L8 (160, 155) -> (160, 180)
  line L9 (185, 155) -> (471.7882, -254.576)
  line L10 (471.7882, -254.576) -> (451.3094, -268.9154)
  line L11 (160, 155) -> (451.3094, -268.9154)
  dimension "d208" = 25
  dimension "d209" = 300
  dimension "d210" = 500
  dimension "d211" = 55
  dimension "d212" = 25
  constraint horizontal L5
  constraint vertical L6
  constraint horizontal L7
  constraint vertical L8
  constraint coincident L4 L5.start
  constraint perpendicular L9 L10
  measures "d208" distance of L5.start L5.end
  measures "d209" distance of L2 L6
  measures "d210" distance of L6.end L9.end
  measures "d211" angle of L1 L9
  measures "d212" distance of L9.end L10.end
extrude "Extrude12" add sketch "Sketch23" against normal blind 25 contours L1 L7 L9 L10 L11 bodies 9 in component "bin case (1)"
sketch "Sketch24" plane through (0, 475, 0) normal (0, 1, 0) x (-1, 0, 0)
  line L0 (-1040.0675, 825) -> (-1040.0675, 0)
  line L1 (-1040.0675, 0) -> (484.9325, 0)
  line L2 (484.9325, 0) -> (484.9325, 825)
  line L3 (484.9325, 825) -> (-1040.0675, 825)
  line L4 (-290.0675, 25) -> (-640.0675, 25)
  line L5 (-640.0675, 25) -> (-640.0675, 800)
  line L6 (-640.0675, 800) -> (-290.0675, 800)
  line L7 (-290.0675, 800) -> (-290.0675, 25)
  line L8 (459.9325, 25) -> (109.9325, 25)
  line L9 (109.9325, 25) -> (109.9325, 800)
  line L10 (109.9325, 800) -> (459.9325, 800)
  line L11 (459.9325, 800) -> (459.9325, 25)
  line L12 (-265.0675, 25) -> (-265.0675, 800)
  line L13 (-265.0675, 800) -> (84.9325, 800)
  line L14 (84.9325, 800) -> (84.9325, 25)
  line L15 (84.9325, 25) -> (-265.0675, 25)
  line L16 (-1015.0675, 25) -> (-1015.0675, 800)
  line L17 (-1015.0675, 800) -> (-665.0675, 800)
  line L18 (-665.0675, 800) -> (-665.0675, 25)
  line L19 (-665.0675, 25) -> (-1015.0675, 25)
  line L20 (459.9325, 800) -> (109.9325, 800)
  line L21 (109.9325, 800) -> (109.9325, 825)
  line L22 (109.9325, 825) -> (459.9325, 825)
  line L23 (459.9325, 825) -> (459.9325, 800)
  line L24 (84.9325, 800) -> (-265.0675, 800)
  line L25 (-265.0675, 800) -> (-265.0675, 825)
  line L26 (-265.0675, 825) -> (84.9325, 825)
  line L27 (84.9325, 825) -> (84.9325, 800)
  line L28 (-290.0675, 800) -> (-640.0675, 800)
  line L29 (-640.0675, 800) -> (-640.0675, 825)
  line L30 (-640.0675, 825) -> (-290.0675, 825)
  line L31 (-290.0675, 825) -> (-290.0675, 800)
  line L32 (-665.0675, 800) -> (-1015.0675, 800)
  line L33 (-1015.0675, 800) -> (-1015.0675, 825)
  line L34 (-1015.0675, 825) -> (-665.0675, 825)
  line L35 (-665.0675, 825) -> (-665.0675, 800)
  constraint horizontal L20
  constraint vertical L21
  constraint horizontal L22
  constraint vertical L23
  constraint coincident L3 L21.end
  constraint coincident L10.end L11.start
  constraint horizontal L24
  constraint vertical L25
  constraint horizontal L26
  constraint vertical L27
  constraint coincident L3 L25.end
  constraint coincident L13.end L14.start
  constraint horizontal L28
  constraint vertical L29
  constraint horizontal L30
  constraint vertical L31
  constraint coincident L3 L29.end
  constraint coincident L6.end L7.start
  constraint horizontal L32
  constraint vertical L33
  constraint horizontal L34
  constraint vertical L35
  constraint coincident L3 L33.end
  constraint coincident L17.end L18.start
extrude "Extrude13" cut sketch "Sketch24" against normal blind 25 contours L3 L17 L32 L33 L34 L35 | L3 L6 L28 L29 L30 L31 | L3 L10 L20 L21 L22 L23 | L3 L13 L24 L25 L26 L27 bodies 9 in component "bin case (1)"
sketch "Sketch25" plane through (0, 0, 875) normal (0, 0, -1) x (1, 0, 0)
  line L0 (-460, 180) -> (-460, 155)
  line L1 (-460, 155) -> (-185, 155)
  line L2 (-185, 155) -> (-471.7882, -254.576)
  line L3 (-471.7882, -254.576) -> (-451.3094, -268.9154)
  line L4 (-451.3094, -268.9154) -> (-160, 155)
  line L5 (-160, 155) -> (1015, 155)
  line L6 (1015, 155) -> (1015, 180)
  line L7 (1015, 180) -> (-460, 180)
  line L8 (-160, 155) -> (-164.1208, 157.8318)
  line L9 (-164.1208, 157.8318) -> (-455.4052, -266.0475)
  line L10 (-455.4052, -266.0475) -> (-451.3094, -268.9154)
  line L11 (-451.3094, -268.9154) -> (-160, 155)
  dimension "d219" = 5
  dimension "d220" = 5
  constraint coincident L4.end L5.start
  constraint perpendicular L4 L8
  constraint coincident L3 L9.end
  constraint coincident L3.end L4.start
  measures "d219" distance of L4.end L8.end
  measures "d220" distance of L3.end L9.end
sketch "Sketch26" plane through (-274.8252, 392.491, 0) normal (-0.573576, 0.819152, 0) x (-0.819152, -0.573576, 0)
  line L0 (240.4475, 900) -> (215.4475, 900)
  line L1 (215.4475, 900) -> (215.4475, 875)
  line L2 (215.4475, 875) -> (240.4475, 875)
  line L3 (240.4475, 875) -> (240.4475, 900)
extrude "Extrude14" add sketch "Sketch25" along normal blind 44 contours L3 L4 L8 L9 L10 L11 bodies 9 in component "bin case (1)"
sketch "Sketch27" plane through (0, -155, 0) normal (0, 1, 0) x (-1, 0, 0)
  line L0 (160, 875) -> (160, 900)
  line L1 (160, 900) -> (-1040, 900)
  line L2 (-1040, 900) -> (-1040, 825)
  line L3 (-1040, 825) -> (-1220, 825)
  line L4 (-1220, 825) -> (-1250.0621, 808.2988)
  arc A0 (-1248.0189, 784.434) -> (-1250.0621, 808.2988) centre (-1265, 795) ccw
  line L5 (-1248.0189, 784.434) -> (-1220, 800)
  line L6 (-1220, 800) -> (-1040, 800)
  line L7 (-1040, 800) -> (-1040, 25)
  line L8 (-1040, 25) -> (-1015, 25)
  line L9 (-1015, 25) -> (-1015, 800)
  line L10 (-1015, 800) -> (-290, 800)
  line L11 (-290, 800) -> (-290, 25)
  line L12 (-290, 25) -> (-265, 25)
  line L13 (-265, 25) -> (-265, 800)
  line L14 (-265, 800) -> (460, 800)
  line L15 (460, 800) -> (460, 25)
  line L16 (460, 25) -> (485, 25)
  line L17 (485, 25) -> (485, 800)
  line L18 (485, 800) -> (486, 800)
  line L19 (486, 800) -> (518.7278, 783.3022)
  arc A1 (519.6212, 807.8463) -> (518.7278, 783.3022) centre (534.95, 795) ccw
  line L20 (519.6212, 807.8463) -> (486, 825)
  line L21 (486, 825) -> (485, 825)
  line L22 (485, 825) -> (485, 875)
  line L23 (485, 875) -> (485, 900)
  line L24 (485, 900) -> (185, 900)
  line L25 (185, 900) -> (185, 875)
  line L26 (185, 875) -> (460, 875)
  line L27 (460, 875) -> (460, 825)
  line L28 (460, 825) -> (-1015, 825)
  line L29 (-1015, 825) -> (-1015, 875)
  line L30 (-1015, 875) -> (160, 875)
  line L31 (225, 900) -> (250, 900)
  line L32 (250, 900) -> (250, 875)
  line L33 (250, 875) -> (225, 875)
  line L34 (225, 875) -> (225, 900)
  dimension "d223" = 25
  dimension "d224" = 40
  constraint horizontal L31
  constraint vertical L32
  constraint horizontal L33
  constraint vertical L34
  constraint coincident L26 L32.end
  constraint coincident L24 L31.start
  measures "d223" distance of L32 L34
  measures "d224" distance of L24.end L34
extrude "Extrude15" add sketch "Sketch27" along normal blind 94 contours L24 L26 L31 L32 L33 L34 bodies 9 in component "bin case (1)"
sketch "Sketch1 (9)" plane through (-459.9325, 0, 0) normal (1, 0, 0) x (0, 1, 0) in component "case lock"
  line L0 (100, 800) -> (450, 800)
  line L1 (450, 800) -> (450, 25)
  line L2 (450, 25) -> (475, 25)
  line L3 (475, 25) -> (475, 825)
  line L4 (475, 825) -> (100, 825)
  line L5 (100, 825) -> (100, 800)
  line L6 (450, 800) -> (475, 800)
  line L7 (475, 800) -> (475, 825)
  line L8 (475, 825) -> (450, 825)
  line L9 (450, 825) -> (450, 800)
  constraint horizontal L6
  constraint vertical L7
  constraint horizontal L8
  constraint vertical L9
  constraint coincident L3.end L4.start
  constraint coincident L0.end L1.start
extrude "Extrude1'''''''" add sketch "Sketch1 (9)" along normal blind 345 separate body contours L3 L4 L6 L7 L8 L9 makes body 19 in component "case lock"
sketch "Sketch28" plane through (0, -180, 0) normal (0, -1, 0) x (1, 0, 0)
  line L0 (1015, 875) -> (1015, 825)
  line L1 (1015, 825) -> (-460, 825)
  line L2 (-460, 825) -> (-460, 875)
  line L3 (-460, 875) -> (1015, 875)
  line L4 (1040, 900) -> (-460, 900)
  line L5 (-460, 900) -> (-485, 900)
  line L6 (-485, 900) -> (-485, 875)
  line L7 (-485, 875) -> (-485, 825)
  line L8 (-485, 825) -> (-486, 825)
  line L9 (-486, 825) -> (-519.6212, 807.8463)
  arc A0 (-519.6212, 807.8463) -> (-535, 775.0001) centre (-534.95, 795) ccw
  line L10 (-535, 775.0001) -> (-535, 775)
  line L11 (-535, 775) -> (-534.9999, 775.0001)
  arc A1 (-534.9999, 775.0001) -> (-518.7278, 783.3022) centre (-534.95, 795) ccw
  line L12 (-518.7278, 783.3022) -> (-486, 800)
  line L13 (-486, 800) -> (-485, 800)
  line L14 (-485, 800) -> (-485, 0)
  line L15 (-485, 0) -> (1040, 0)
  line L16 (1040, 0) -> (1040, 800)
  line L17 (1040, 800) -> (1220, 800)
  line L18 (1220, 800) -> (1248.0189, 784.434)
  arc A2 (1248.0189, 784.434) -> (1250.0621, 808.2988) centre (1265, 795) ccw
  line L19 (1250.0621, 808.2988) -> (1220, 825)
  line L20 (1220, 825) -> (1040, 825)
  line L21 (1040, 825) -> (1040, 900)
  line L22 (-460, 800) -> (265, 800)
  line L23 (265, 800) -> (265, 25)
  line L24 (265, 25) -> (-460, 25)
  line L25 (-460, 25) -> (-460, 800)
  line L26 (290, 800) -> (1015, 800)
  line L27 (1015, 800) -> (1015, 25)
  line L28 (1015, 25) -> (290, 25)
  line L29 (290, 25) -> (290, 800)
  line L30 (1015, 865) -> (1040, 865)
  line L31 (1040, 865) -> (1040, 840)
  line L32 (1040, 840) -> (1015, 840)
  line L33 (1015, 840) -> (1015, 865)
  dimension "d253" = 25
  dimension "d254" = 15
  constraint horizontal L30
  constraint vertical L31
  constraint horizontal L32
  constraint vertical L33
  constraint coincident L0 L30.start
  measures "d253" distance of L30.start L32.end
  measures "d254" distance of L1 L32
extrude "Extrude16" add sketch "Sketch28" along normal blind 350 contours L0 L21 L30 L31 L32 L33 bodies 9 in component "bin case (1)"
sketch "Sketch1 (10)" plane through (1015, 0, 0) normal (-1, 0, 0) x (0, -1, 0) in component "mortor b2"
  line L0 (180, 875) -> (155, 875)
  line L1 (155, 875) -> (155, 825)
  line L2 (155, 825) -> (180, 825)
  line L3 (180, 825) -> (180, 840)
  line L4 (180, 840) -> (530, 840)
  line L5 (530, 840) -> (530, 865)
  line L6 (530, 865) -> (180, 865)
  line L7 (180, 865) -> (180, 875)
  circle A0 centre (195, 872.5) radius 7.5
  dimension "d263" = 15
  dimension "d264" = 7.5
  dimension "d265" = 15
  measures "d263" diameter of A0
  measures "d264" distance of L6 A0.centre
  measures "d265" distance of L7 A0.centre
extrude "Extrude1''''''''" add sketch "Sketch1 (10)" along normal blind 5 and the other way blind 30 separate body contours A0 makes body 20 in component "mortor b2"
sketch "Sketch2 (6)" plane through (1010, 0, 0) normal (-1, 0, 0) x (0, -1, 0) in component "mortor b2"
  circle A0 centre (195, 872.5) radius 7.5
  circle A1 centre (195, 872.5) radius 13
  dimension "d266" = 26
  constraint concentric A0 A1
  measures "d266" diameter of A1
extrude "Extrude2'''''''" add sketch "Sketch2 (6)" along normal blind 35 contours A0 | A1 bodies 20 in component "mortor b2"